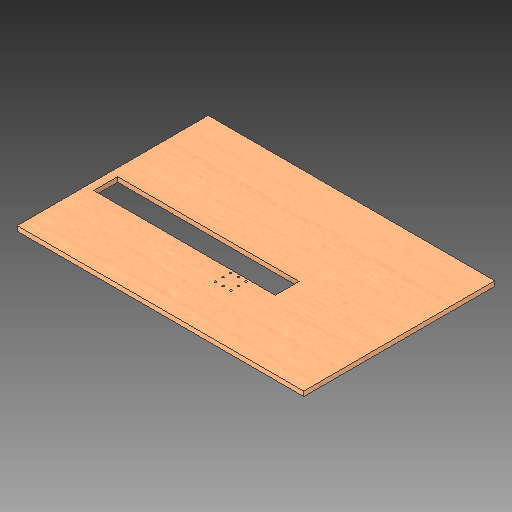
# Autodesk Inventor part: face-lateral
Saved by Autodesk Inventor 2019 (Build 230136000, 136)
## iProperties
Created: 2018-04-02
Part Number: face-lateral
Material: Générique
Document SubType Name: Modeling
Designer: franc
Density: 1 g/cm^3
Appearance: Par défaut
Author: franc
Autodesk Inventor part; units mm, degrees
ref_plane "YZ Plane" through (0, 0, 0) normal (1, 0, 0) x (0, 1, 0)
ref_plane "XZ Plane" through (0, 0, 0) normal (0, 1, 0) x (-1, 0, 0)
ref_plane "XY Plane" through (0, 0, 0) normal (0, 0, 1) x (1, 0, 0)
sketch "Esquisse1" plane through (0, 0, 0) normal (0, 1, 0) x (-1, 0, 0)
  line L0 (98.2051, 94.359) -> (-201.7949, 94.359)
  line L1 (-201.7949, 94.359) -> (-201.7949, -105.641)
  line L2 (-201.7949, -105.641) -> (98.2051, -105.641)
  line L3 (98.2051, -105.641) -> (98.2051, 94.359)
  point P0 (0, 0)
  dimension "d0" = 200
  dimension "d1" = 300
  constraints: 8 end point, 2 parallel, 1 horizontal, 1 perpendicular
  measures "d0" distance of L2.end L0.start
  measures "d1" distance of L1.end L2.end
extrude "Extrusion1" add sketch "Esquisse1" along normal blind 5
sketch "Esquisse2" plane through (0, 5, 0) normal (0, 1, 0) x (1, 0, 0)
  line L0 (89.9575, -12.359) -> (-80.036, -12.359) projected
  line L1 (89.9575, -7.359) -> (-80.036, -7.359) projected
  line L2 (-80.036, -12.359) -> (-80.036, -7.359) projected
  line L3 (89.9575, -12.359) -> (89.9575, -7.359) projected
  line L4 (-90.036, -22.359) -> (99.9575, -22.359)
  line L5 (99.9575, -22.359) -> (99.9575, 2.641)
  line L6 (99.9575, 2.641) -> (-90.036, 2.641)
  line L7 (-90.036, 2.641) -> (-90.036, -22.359)
  point P0 (0, 0)
  dimension "d4" = 10
  dimension "d5" = 10
  dimension "d6" = 10
  dimension "d7" = 10
  constraints: 8 end point, 2 parallel, 1 horizontal, 1 perpendicular
  measures "d4" distance between parallel lines of L4 L0
  measures "d5" distance between parallel lines of L6 L1
  measures "d6" distance between parallel lines of L7 L2
  measures "d7" distance between parallel lines of L3 L5
extrude "Extrusion2" cut sketch "Esquisse2" against normal through all contours L0 L2 L1 L3 | L7 L6 L5 L4
sketch "Esquisse3" plane through (0, 0, 0) normal (0, -1, 0) x (1, 0, 0)
  circle A0 centre (56.2949, 33.359) radius 1 projected
  line L0 (57.2949, 15.359) -> (55.2949, 15.359) projected
  circle A1 centre (56.2949, 41.359) radius 1 projected
  circle A2 centre (64.2949, 41.359) radius 1 projected
  circle A3 centre (72.2949, 33.359) radius 1 projected
  circle A4 centre (72.2949, 41.359) radius 1 projected
  circle A5 centre (72.2949, 25.359) radius 1 projected
  circle A6 centre (64.2949, 25.359) radius 1 projected
  circle A7 centre (56.2949, 25.359) radius 1 projected
  point P0 (0, 0)
extrude "Extrusion3" cut sketch "Esquisse3" against normal through all
